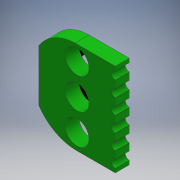
# Autodesk Inventor part: Encoder_optico
Saved by Autodesk Inventor 2017 (Build 210142000, 142)
## iProperties
Created: 2016-07-29
Part Number: Encoder_optico
Material: Generic
Document SubType Name: Modeling
Designer: ANDRES
Density: 1 g/cm^3
Appearance: Default
Author: ANDRES
Autodesk Inventor part; units mm, degrees
ref_plane "YZ Plane" through (0, 0, 0) normal (1, 0, 0) x (0, 1, 0)
ref_plane "XZ Plane" through (0, 0, 0) normal (0, 1, 0) x (-1, 0, 0)
ref_plane "XY Plane" through (0, 0, 0) normal (0, 0, 1) x (1, 0, 0)
sketch "Sketch1" plane through (0, 0, 0) normal (0, 1, 0) x (-1, 0, 0)
  line L0 (-4.8, -5.8) -> (0.1217, -5.8)
  line L1 (4.8, -3.25) -> (4.8, 3.25)
  line L2 (0.2433, 5.8) -> (-4.8, 5.8)
  line L3 (-4.8, 5.8) -> (-4.8, -5.8)
  line L4 (-4.8, -5.8) -> (4.8, 5.8) construction
  line L5 (4.8, -5.8) -> (-4.8, 5.8) construction
  line L6 (4.8, 0) -> (4.8, 3.25) construction
  arc A0 (4.8, 3.25) -> (0, 5.8) centre (0.1217, 0.2363) ccw
  line L7 (4.8, 0) -> (4.8, -3.25) construction
  arc A1 (0, -5.8) -> (4.8, -3.25) centre (0.0608, -0.1218) ccw
  circle A2 centre (0, 3.94) radius 1.5
  circle A3 centre (0, 0.08) radius 1.5
  circle A4 centre (0, -3.78) radius 1.5
  arc A5 (-4.8, 4.3) -> (-4.8, 5.3) centre (-4.8, 4.8) ccw
  arc A6 (-4.8, 2.38) -> (-4.8, 3.38) centre (-4.8, 2.88) ccw
  arc A7 (-4.8, 0.46) -> (-4.8, 1.46) centre (-4.8, 0.96) ccw
  arc A8 (-4.8, -1.46) -> (-4.8, -0.46) centre (-4.8, -0.96) ccw
  arc A9 (-4.8, -3.38) -> (-4.8, -2.38) centre (-4.8, -2.88) ccw
  arc A10 (-4.8, -5.3) -> (-4.8, -4.3) centre (-4.8, -4.8) ccw
  line L8 (-4.8, 3.38) -> (-4.8, 2.38)
  line L9 (-4.8, 1.46) -> (-4.8, 0.46)
  line L10 (-4.8, -0.46) -> (-4.8, -1.46)
  line L11 (-4.8, -2.38) -> (-4.8, -3.38)
  line L12 (-4.8, -4.3) -> (-4.8, -5.3)
  point P0 (0, 0)
  dimension "d0" = 9.6
  dimension "d1" = 11.6
  dimension "d2" = 3.25
  dimension "d3" = 3.25
  dimension "d4" = 3
  dimension "d5" = 1.86
  dimension "d8" = 3.86
  dimension "d13" = 1
  dimension "d14" = 1
  dimension "d17" = 1.92
  dimension "d32" = 4.8
  constraints: 26 end point, 18 point on circle, 11 centre point, 5 collinear, 5 point on line, 3 midpoint, 2 parallel, 2 vertical, 1 horizontal, 1 perpendicular, 24 other
  measures "d0" distance of L2.end L4.end
  measures "d1" distance of L4.end L5.start
  measures "d2" distance of L1.end L6.start
  measures "d3" distance of L1.start L6.start
  measures "d4" diameter of A2
  measures "d5" distance from line of A2.centre L2
  measures "d8" distance of A2.centre A3.centre
  measures "d13" diameter of A5
  measures "d14" distance from line of L2 A5.centre
  measures "d17" distance of A5.centre A6.centre
  measures "d32" distance from line of L3 A2.centre
extrude "Extrusion2" add sketch "Sketch1" along normal blind 1.75 contours L3 A10 A9 A8 A7 A6 A5 L2 A0 L1 A1 L0
sketch "Sketch2" plane through (0, 1.75, 0) normal (0, 1, 0) x (1, 0, 0)
  line L0 (-1.7477, -2.7588) -> (-2.9764, -3.6192)
  line L1 (-2.9764, -3.6192) -> (-4.4104, -1.5713)
  line L2 (-4.4104, -1.5713) -> (-3.1816, -0.7109)
  line L3 (-3.1816, -0.7109) -> (-1.7477, -2.7588)
  line L4 (-4.55, -1.3) -> (-2.55, -4.3) construction
  line L5 (-2.55, -1.3) -> (-4.55, -4.3) construction
  line L6 (-0.2433, -5.8) -> (4.8, -5.8) projected
  line L7 (0, -5.8) -> (0, 5.8)
  line L8 (4.8, 5.8) -> (-0.1217, 5.8) projected
  line L9 (-4.8, 3.25) -> (-4.8, -3.25) projected
  line L10 (-4.8, 0) -> (4.8, 0) construction
  line L11 (-1.7477, 2.7588) -> (-2.9764, 3.6192)
  line L12 (-2.9764, 3.6192) -> (-4.4104, 1.5713)
  line L13 (-4.4104, 1.5713) -> (-3.1816, 0.7109)
  line L14 (-3.1816, 0.7109) -> (-1.7477, 2.7588)
  point P0 (0, 0)
  point P1 (-3.55, -2.8)
  point P2 (-3.55, -2.8)
  dimension "d26" = 1.5
  dimension "d27" = 2.5
  dimension "d28" = 1.25
  dimension "d29" = 3
  constraints: 24 end point, 4 midpoint, 4 symmetric about line, 3 point on line, 2 parallel, 1 horizontal, 1 perpendicular, 1 vertical
  measures "d26" distance of L1.end L2.end
  measures "d27" distance of L0.end L1.end
  measures "d28" distance from line of L9 point (-3.55, -2.8)
  measures "d29" distance from line of L6 point (-3.55, -2.8)
extrude "Extrusion3" add sketch "Sketch2" along normal blind 1.5
body "Solid2"
